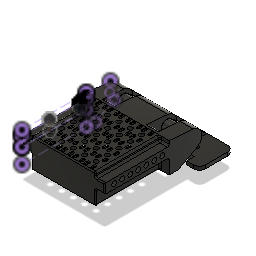
_Shell Mount.6282c432-1834-4d19-9b96-cbeaaebe9f8f (Autodesk Fusion 360 design; units mm, degrees)
Autodesk Fusion 360 part; units mm, degrees
note: some values were not read from the file. Chosen so that the rebuilt part matches the saved one: that a step has no effect; which face or edge a step refers to; which pieces of a blend or face edit are solid. Set by a fixed rule: which sketch regions a step uses.
ref_plane "WorkPlane2" through (12.125, 0, 0) normal (0, 0.422618, 0.906308) x (1, 0, 0)
sketch "Sketch1" plane through (0, 0, 0) normal (0, 0.422618, 0.906308) x (1, 0, 0)
  line L0 (0, 0) -> (94.7, 0)
  line L1 (94.7, 0) -> (94.7, 29.7)
  line L2 (94.7, 29.7) -> (0, 29.7)
  line L3 (0, 29.7) -> (0, 0)
  circle A0 centre (17.35, 14.85) radius 2.05
  line L4 (47.35, 29.7) -> (47.35, 0)
  line L5 (17.35, 14.85) -> (17.35, 29.7) construction
  line L6 (17.35, 14.85) -> (17.35, 0) construction
  circle A1 centre (77.35, 14.85) radius 2.05
  dimension "d1" = 94.7
  dimension "d2" = 29.7
  dimension "d3" = 60
  dimension "d4" = 4.1
  constraint horizontal L0
  constraint vertical L1
  constraint horizontal L2
  constraint vertical L3
  constraint coincident L0.start L3.end
  constraint midpoint L2 L4.start
  constraint midpoint L0 L4.end
  constraint coincident A0.centre L5.start
  constraint coincident L2 L5.end
  constraint perpendicular L2 L5
  constraint coincident L0 L6.end
  constraint perpendicular L0 L6
  constraint equal L5 L6
  constraint symmetric A0 L4 A1
  measures "d1" distance of L1.end L2.end
  measures "d2" distance of L0.end L1.end
  measures "d3" distance of A0.centre A1.centre
  measures "d4" diameter of A0
extrude "Extrude3" add sketch "Sketch1" along normal blind 3 contours L0 L2 L3 L4 makes body 1
ref_plane "WorkPlane3" through (23.675, 14.0926, -4.9164) normal (1, 0, 0) x (0, 0.906308, -0.422618)
ref_plane "WorkPlane6" through (23.175, 14.0926, -4.9164) normal (1, 0, 0) x (0, 0.906308, -0.422618)
sketch "Sketch3" plane through (23.175, 0, 0) normal (1, 0, 0) x (0, 0, -1)
  circle A0 centre (-12.3878, 11.2934) radius 5
  line L0 (12.5518, 26.9173) -> (9.8328, 28.1852)
  line L1 (9.8328, 28.1852) -> (-2.7189, 1.2679)
  line L2 (0, 0) -> (-2.7189, 1.2679)
  line L3 (12.5518, 26.9173) -> (0, 0)
  line L4 (-14.6517, 15.7515) -> (9.8328, 28.1852)
  line L5 (-14.5009, 6.7619) -> (-2.7189, 1.2679)
  circle A1 centre (-12.3878, 11.2934) radius 5.3
  line L6 (-1.75, 0) -> (-22.5, 0)
  line L7 (-2.7189, 1.2679) -> (-3.3101, 0)
  circle A2 centre (-12.3878, 11.2934) radius 8.3
  line L8 (-8.4967, 3.9621) -> (-24.8293, -4.7066)
  line L9 (-11.7076, 19.5655) -> (-32.7189, 21.2934)
  line L10 (-24.8293, -4.7066) -> (-32.7189, -4.7066)
  line L11 (-32.7189, -4.7066) -> (-32.7189, 21.2934)
  arc A3 (-30.1359, 21.081) -> (-24.8293, -4.7066) centre (-12.3878, 11.2934) ccw
  arc A4 (-26.8354, 20.8096) -> (-21.9042, -3.154) centre (-12.3878, 11.2934) ccw
  point P0 (-2.7189, 1.2679)
  point P1 (-8.4967, 3.9621)
  dimension "d13" = 10
  dimension "d14" = 13
  dimension "d21" = 0.3
  dimension "d24" = 3
  dimension "d27" = 26
  dimension "d31" = 16
  dimension "d32" = 3
  dimension "d34" = 30
  dimension "d95" = 9
  constraint coincident A0 L4.start
  constraint coincident L0.end L1.start
  constraint coincident A0 L5.start
  constraint coincident P0 L1.end
  constraint tangent A0 L5
  constraint tangent A0 L4
  constraint collinear L2 L5
  constraint concentric A0 A1
  constraint coincident L6 L7.end
  constraint perpendicular L2 L7
  constraint concentric A0 A2
  constraint coincident A2 P1
  constraint tangent A2 L8
  constraint coincident A2 L9.start
  constraint tangent A2 L9
  constraint perpendicular L10 L11
  constraint parallel L6 L10
  constraint coincident L9 A3.start
  constraint coincident A0.centre A1.centre
  constraint coincident L5 P1
  constraint coincident P1 L8.start
  constraint coincident L9 A4.start
  constraint coincident L8 A4.end
  measures "d13" diameter of A0
  measures "d14" distance of A0.centre L1
  measures "d21" distance of A0 A1
  measures "d24" distance of A1 A2
  measures "d27" distance of L9.end L10.end
  measures "d31" distance of A0.centre L10
  measures "d32" distance of L1 L3
  measures "d34" distance of L11 P0
  measures "d95" distance of A2 A4
extrude "Extrude4" add sketch "Sketch3" along normal blind 10 contours A0 L4 L5 A1 | L4 L5 A1 A2 | L1 L4 L5 A2 picked at (-12.8199, 6.2206) picked at (-8.6605, 17.5523) bodies 1
extrude "Extrude5" add sketch "Sketch3" along normal blind 10 and the other way blind 11 draft -45 separate body contours A0 makes body 2
extrude "Extrude6" add sketch "Sketch3" against normal blind 8 draft -45 separate body contours A0 | A0 L4 L5 A1 | A0 L4 L5 A1 makes body 3
extrude "Extrude7" add 1 faces at (33.175, 10.6437, 14.8692) along direction (1, 0, 0) blind 7.4 draft -45 on bodies 2 bodies 2 3 1
ref_plane "WorkPlane4" through (28.175, 14.7265, 2.4094) normal (-1, 0, 0) x (0, 0, 1)
extrude "Extrude8" add sketch "Sketch3" along normal blind -12 and the other way blind 0.2 separate body contours A0 | A0 L4 L5 A1 | A0 L4 L5 A1 | L4 L5 A1 A2 | L4 L5 A1 A2 | A2 L8 L9 A4 | L8 L9 A3 A4 | L9 L10 L11 A3 makes body 4
combine "Combine1" operation cut target body 4 tool bodies 3
mirror "Mirror1" about plane through (28.175, 14.7265, 2.4094) normal (-1, 0, 0) of bodies 4 makes body 5
extrude "Extrude14" add 1 faces at (45.175, 12.0508, 23.0853) along direction (1, 0, 0) blind 2.175 on bodies 5 bodies 5
mirror "Mirror3" [no effect]
extrude "Extrude9" add sketch "Sketch3" along normal blind 23.675 and the other way blind 6 contours L8 L9 A3 A4 | L9 L10 L11 A3 bodies 4 5
sketch "Sketch7" plane through (0, 0, 32.7189) normal (0, 0, 1) x (1, 0, 0)
  line L0 (47.35, 21.2934) -> (11.175, 21.2934)
  line L1 (11.175, 21.2934) -> (11.175, -4.7066)
  line L2 (11.175, -4.7066) -> (47.35, -4.7066)
  line L3 (47.35, -4.7066) -> (47.35, 21.2934)
  line L4 (11.175, 17.0915) -> (19.175, 17.0915)
  line L5 (11.175, 8.4915) -> (19.175, 8.4915)
  line L6 (19.175, 17.0915) -> (19.175, 21.2934)
  line L7 (19.175, 8.4915) -> (19.175, -4.7066)
  dimension "d96" = 8.6
  dimension "d97" = 8
  constraint coincident L1 L4.start
  constraint perpendicular L3 L4
  constraint coincident L1 L5.start
  constraint perpendicular L1 L5
  constraint coincident L0 L6.end
  constraint perpendicular L0 L6
  constraint coincident L2 L7.end
  constraint perpendicular L2 L7
  constraint collinear L6 L7
  measures "d96" distance of L4 L5
  measures "d97" distance of L4.start L4.end
extrude "Extrude15" add sketch "Sketch7" along normal blind 56.3 contours L0 L1 L2 L3 L4 L5 L6 L7 bodies 4
sketch "Sketch8" plane through (11.175, 0, 0) normal (-1, 0, 0) x (0, 0, 1)
  line L0 (32.7189, -4.7066) -> (32.7189, 8.4915) construction
  line L1 (32.7189, 21.2934) -> (11.7076, 19.5655) construction
  arc A0 (11.7076, 19.5655) -> (8.4967, 3.9621) centre (12.3878, 11.2934) ccw
  line L2 (8.4967, 3.9621) -> (24.8293, -4.7066)
  line L3 (24.8293, -4.7066) -> (32.7189, -4.7066) construction
  line L4 (32.7189, 8.4915) -> (89.0189, 8.4915) construction
  line L5 (89.0189, 8.4915) -> (89.0189, 17.0915) construction
  line L6 (89.0189, 17.0915) -> (32.7189, 17.0915) construction
  line L7 (32.7189, 17.0915) -> (32.7189, 21.2934) construction
  arc A1 (11.7076, 19.5655) -> (8.4967, 3.9621) centre (12.3878, 11.2934) ccw construction
  line L8 (8.4967, 3.9621) -> (24.8293, -4.7066) construction
  line L9 (24.8293, -4.7066) -> (32.7189, -4.7066) construction
  line L10 (32.7189, -4.7066) -> (32.7189, 8.4915) construction
  line L11 (32.7189, 8.4915) -> (89.0189, 8.4915) construction
  line L12 (89.0189, 8.4915) -> (89.0189, 17.0915) construction
  line L13 (89.0189, 17.0915) -> (32.7189, 17.0915) construction
  line L14 (32.7189, 17.0915) -> (32.7189, 21.2934) construction
  line L15 (32.7189, 21.2934) -> (11.7076, 19.5655) construction
  line L16 (32.7189, 21.2934) -> (32.7189, 17.0915) construction
  line L17 (32.7189, 17.0915) -> (89.0189, 17.0915) construction
  line L18 (89.0189, 17.0915) -> (89.0189, 21.2934) construction
  line L19 (89.0189, 21.2934) -> (32.7189, 21.2934) construction
  line L20 (32.7189, 8.4915) -> (32.7189, -4.7066) construction
  line L21 (32.7189, -4.7066) -> (89.0189, -4.7066) construction
  line L22 (89.0189, -4.7066) -> (89.0189, 8.4915) construction
  line L23 (89.0189, 8.4915) -> (32.7189, 8.4915) construction
  circle A2 centre (38.7189, 12.7915) radius 2.1
  line L24 (64.7189, 8.4915) -> (64.7189, 17.0915) construction
  line L25 (38.7189, 12.7915) -> (38.7189, 17.0915) construction
  line L26 (38.7189, 12.7915) -> (38.7189, 8.4915) construction
  line L27 (32.7189, 8.4915) -> (32.7189, 17.0915) construction
  dimension "d108" = 4.2
  dimension "d168" = 6
  constraint coincident L11 L24.start
  constraint coincident L13 L24.end
  constraint perpendicular L13 L24
  constraint coincident A2.centre L25.start
  constraint coincident L13 L25.end
  constraint perpendicular L13 L25
  constraint coincident L11 L26.end
  constraint perpendicular L11 L26
  constraint coincident L0.end L4.start
  constraint coincident L6.end L7.start
  measures "d108" diameter of A2
  measures "d168" distance of A2.centre L27
extrude "Extrude16" cut sketch "Sketch8" against normal blind 10 bodies 4
pattern_linear "R-Pattern1" count 7 spacing 7 along (0, 0, 1) of "Extrude16"
fillet "Fillet4" radius 1.5 8 edges at (19.175, 17.0915, 60.8689) (19.175, 8.4915, 60.8689) (19.175, 21.2934, 60.8689) (19.175, -4.7066, 60.8689) (15.175, 8.4915, 32.7189) (19.175, 1.8924, 32.7189) (19.175, 19.1924, 32.7189) (15.175, 17.0915, 32.7189) on bodies 4
chamfer "Chamfer3" distance 1 angle 45 11 edges at (34.0125, 21.2934, 89.0189) (19.6143, 20.8541, 89.0189) (19.175, 19.1924, 89.0189) (18.7357, 17.5308, 89.0189) (14.425, 17.0915, 89.0189) (34.0125, -4.7066, 89.0189) (14.425, 8.4915, 89.0189) (18.7357, 8.0521, 89.0189) (19.175, 1.8924, 89.0189) (19.6143, -4.2672, 89.0189) (11.175, 12.7915, 89.0189) on bodies 4
mirror "Mirror4" about plane through (47.35, 26.9173, -12.5518) normal (1, 0, 0) of bodies 4 2 merged
sketch "Sketch9" plane through (0, 21.2934, 0) normal (0, 1, 0) x (-1, 0, 0)
  line L0 (-76.6231, 32.7189) -> (-18.0769, 32.7189)
  circle A0 centre (-27.35, 40.3689) radius 1.95
  line L1 (-23.6, 33.6189) -> (-25.1, 33.6189)
  line L2 (-23.6, 37.1189) -> (-25.1, 33.6189) construction
  line L3 (-25.1, 33.6189) -> (-25.1, 37.1189)
  line L4 (-25.1, 37.1189) -> (-23.6, 33.6189) construction
  line L5 (-23.6, 37.1189) -> (-23.6, 33.6189)
  line L6 (-27.35, 40.3689) -> (-27.35, 32.7189) construction
  line L7 (-25.1, 37.1189) -> (-23.6, 37.1189)
  line L8 (-23.6, 33.6189) -> (-23.6, 32.7189) construction
  line L9 (-20.675, 88.0189) -> (-74.025, 88.0189)
  line L10 (-74.025, 88.0189) -> (-74.025, 34.2189)
  spline S0 degree 3 poles (-74.025, 34.2189) (-74.4406, 33.8033) (-74.9478, 33.3131) (-75.6338, 32.9439) (-75.8264, 32.8608) (-76.2254, 32.7481) (-76.4319, 32.7189) (-76.6231, 32.7189) knots 0 0 0 0 0.176344 0.176344 0.233692 0.233692 0.291039 0.291039 0.291039 0.291039
  spline S1 degree 3 poles (-20.675, 34.2189) (-20.2594, 33.8033) (-19.7522, 33.3131) (-19.0662, 32.9439) (-18.8736, 32.8608) (-18.4746, 32.7481) (-18.2681, 32.7189) (-18.0769, 32.7189) knots 0 0 0 0 0.176344 0.176344 0.233692 0.233692 0.291039 0.291039 0.291039 0.291039
  line L11 (-20.675, 34.2189) -> (-20.675, 88.0189)
  line L12 (-47.35, 32.7189) -> (-47.35, 88.0189) construction
  line L13 (-20.675, 60.3689) -> (-74.025, 60.3689) construction
  circle A1 centre (-67.35, 40.3689) radius 1.95
  line L14 (-69.6, 33.6189) -> (-69.6, 37.1189)
  line L15 (-71.1, 37.1189) -> (-69.6, 33.6189) construction
  line L16 (-71.1, 37.1189) -> (-71.1, 33.6189)
  line L17 (-69.6, 37.1189) -> (-71.1, 33.6189) construction
  line L18 (-71.1, 33.6189) -> (-69.6, 33.6189)
  line L19 (-69.6, 37.1189) -> (-71.1, 37.1189)
  line L20 (-71.1, 33.6189) -> (-71.1, 32.7189) construction
  circle A2 centre (-27.35, 80.3689) radius 1.95
  line L21 (-23.6, 83.6189) -> (-23.6, 87.1189)
  line L22 (-23.6, 87.1189) -> (-23.6, 88.0189) construction
  line L23 (-25.1, 87.1189) -> (-25.1, 83.6189)
  line L24 (-23.6, 87.1189) -> (-25.1, 87.1189)
  line L25 (-25.1, 83.6189) -> (-23.6, 83.6189)
  line L26 (-25.1, 83.6189) -> (-23.6, 87.1189) construction
  line L27 (-23.6, 83.6189) -> (-25.1, 87.1189) construction
  line L28 (-20.675, 34.2189) -> (-20.675, 32.7189) construction
  line L29 (-25.1, 36.3689) -> (-25.1, 34.3689)
  arc A3 (-25.1, 34.3689) -> (-23.6, 34.3689) centre (-24.35, 34.3689) ccw
  line L30 (-23.6, 34.3689) -> (-23.6, 36.3689)
  arc A4 (-23.6, 36.3689) -> (-25.1, 36.3689) centre (-24.35, 36.3689) ccw
  line L31 (-24.35, 36.3689) -> (-24.35, 34.3689) construction
  point P0 (-24.35, 35.3689)
  point P1 (-27.35, 40.3689)
  point P2 (-70.35, 35.3689)
  point P3 (-24.35, 85.3689)
  point P4 (-24.35, 35.3689)
  dimension "d129" = 3.5
  dimension "d130" = 1.5
  dimension "d135" = 5
  dimension "d136" = 3
  dimension "d137" = 3.9
  dimension "d170" = 40
  dimension "d171" = 40
  dimension "d172" = 40
  constraint perpendicular L5 L7
  constraint parallel L1 L7
  constraint parallel L3 L5
  constraint coincident P4 L4
  constraint coincident P4 L2
  constraint coincident P1 A0.centre
  constraint coincident L0 L6.end
  constraint perpendicular L0 L6
  constraint parallel L3 L6
  constraint coincident L0 L8.end
  constraint perpendicular L0 L8
  constraint midpoint L0 L12.start
  constraint midpoint L9 L12.end
  constraint coincident L11 L13.start
  constraint coincident L10 L13.end
  constraint perpendicular L10 L13
  constraint midpoint L12 L13
  constraint symmetric L1.start L12 L16.end
  constraint symmetric L1.end L12 L14.start
  constraint symmetric L2.start L12 L15.start
  constraint symmetric L3.end L12 L14.end
  constraint symmetric P4 L12 P2
  constraint symmetric A0 L12 A1
  constraint symmetric L8.end L12 L20.end
  constraint symmetric L1.start L13 L21.end
  constraint symmetric L1.end L13 L23.start
  constraint symmetric L2.start L13 L21.start
  constraint symmetric L3.end L13 L23.end
  constraint symmetric P4 L13 P3
  constraint symmetric A0 L13 A2
  constraint symmetric L8.end L13 L22.end
  constraint coincident S1.start L11.start
  constraint coincident L0 L28.end
  constraint perpendicular L0 L28
  constraint tangent L29 A3
  constraint tangent A3 L30
  constraint parallel L29 L30
  constraint tangent L30 A4
  constraint tangent L29 A4
  constraint parallel L5 L31
  constraint coincident P4 P0
  constraint midpoint L31 P4
  constraint tangent L1 A3
  constraint tangent L3 A3
  measures "d129" distance of L1.end L3.end
  measures "d130" distance of L2.start L3.end
  measures "d135" vertical distance of P1 P4
  measures "d136" horizontal distance of P4 P1
  measures "d137" diameter of A0
  measures "d170" distance of P1 A1.centre
  measures "d171" distance of P1 A2.centre
  measures "d172" distance of P1 A2.centre
revolve "Revolve1" cut sketch "Sketch9" angle 360 about axis through (27.35, 21.2934, 40.3689) along (0, 0, -1) contours L3 L5 L29 A3 L30 A4 bodies 4
extrude "Extrude18" cut sketch "Sketch9" against normal blind 100 contours A0 bodies 4
fillet "Fillet3" radius 0.5 8 edges at (30.35, 21.2934, 33.6189) (29.6, 21.2934, 35.3689) (31.1, 21.2934, 35.3689) (30.35, 21.2934, 37.1189) (25.1, 21.2934, 35.3689) (24.35, 21.2934, 33.6189) (24.35, 21.2934, 37.1189) (23.6, 21.2934, 35.3689) on bodies 4
pattern_linear "R-Pattern3" count 5 spacing 10 along (1, 0, 0) count 6 spacing 10 along (0, 0, 1) of "Revolve1", "Fillet3"
pattern_linear "R-Pattern4" count 5 spacing 10 along (1, 0, 0) count 5 spacing 10 along (0, 0, 1) of "Extrude18"
copy_body "Body->Comp1" bodies 2 removing the originals makes body 6 in component "Component"
copy_body "Body->Comp2" bodies 4 removing the originals makes body 7 in component "Component'"
combine "Combine1'" operation cut target body 6 tool bodies 7 body 7 seen with x (1, 0, 0) y (0, -0.087156, 0.996195) z (0, -0.996195, -0.087156) at (0, 24.6184, 2.217) keep tools in component "Component"
extrude "Extrude1" cut 1 faces at (22.975, 4.2989, 0.2021) along direction (1, 0, 0) blind 0.2 on bodies 6 bodies 6 in component "Component"
extrude "Extrude2" cut 1 faces at (33.375, 4.2989, 0.2021) along direction (-1, 0, 0) blind 0.2 on bodies 6 bodies 6 in component "Component"
extrude "Extrude3'" cut 1 faces at (71.725, 4.2989, 0.2021) along direction (-1, 0, 0) blind 0.2 on bodies 6 bodies 6 in component "Component"
extrude "Extrude4'" cut 1 faces at (61.325, 4.2989, 0.2021) along direction (1, 0, 0) blind 0.2 on bodies 6 bodies 6 in component "Component"
fillet "Fillet1" radius 5 4 edges at (0, 0.6339, 1.3595) (0, 27.5513, -11.1923) (94.7, 0.6339, 1.3595) (94.7, 27.5513, -11.1923) on bodies 6 in component "Component"
fillet "Fillet1'" radius 2.5 4 edges at (66.525, 20.8096, 26.8354) (28.175, 20.8096, 26.8354) (66.525, -3.154, 21.9042) (28.175, -3.154, 21.9042) on bodies 7 in component "Component'"
component "Component" placed x (1, 0, 0) y (0, 0.422618, -0.906308) z (0, 0.906308, 0.422618) at (0, -4.7066, 17.3878)
component "Component'" placed x (1, 0, 0) y (0, 1, 0) z (0, 0, 1) at (0, 0, 0)
equation "d1 = 95 mm - 0.3 mm"
equation "d2 = 30 mm - 0.3 mm"
equation "d8 = 90 deg - 115 deg"
